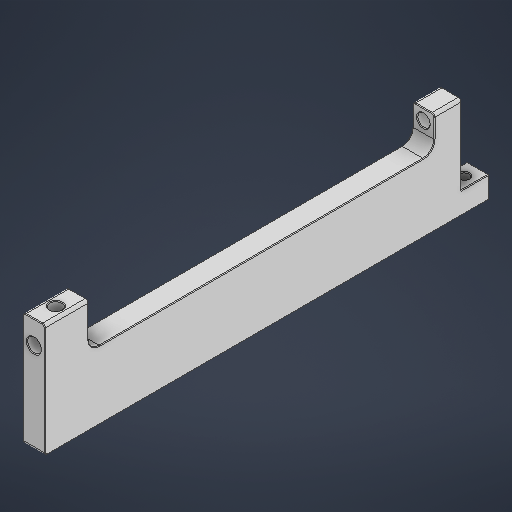
# Autodesk Inventor part: Half-Shaft-Motor
Saved by Autodesk Inventor 2025 (Build 290162010, 162A)
## iProperties
Created: 2025-12-05
Part Number: Half-Shaft-Motor
Material: Generic
Document SubType Name: Modeling
Designer: FizzyApple12
Density: 1 g/cm^3
Appearance: Default
Author: FizzyApple12
Autodesk Inventor part; units mm, degrees
ref_plane "YZ Plane" through (0, 0, 0) normal (1, 0, 0) x (0, 1, 0)
ref_plane "XZ Plane" through (0, 0, 0) normal (0, 1, 0) x (-1, 0, 0)
ref_plane "XY Plane" through (0, 0, 0) normal (0, 0, 1) x (1, 0, 0)
sketch "Sketch1" plane through (0, 0, 0) normal (0, 0, 1) x (1, 0, 0)
  circle A0 centre (0, 0) radius 2.5
  line L0 (-4, -8) -> (4, -8)
  line L1 (4, -8) -> (4, -33)
  line L2 (4, -33) -> (-4, -33)
  line L3 (-4, -33) -> (-4, -8)
  line L4 (0, 0) -> (0, -8) construction
  line L5 (-4, -8) -> (4, -8)
  line L6 (4, -8) -> (4, 4)
  line L7 (4, 4) -> (-4, 4)
  line L8 (-4, 4) -> (-4, -8)
  line L9 (0, 0) -> (0, 4) construction
  line L10 (-4, 4) -> (4, 4)
  line L11 (4, 4) -> (4, 8.5)
  line L12 (4, 8.5) -> (-4, 8.5)
  line L13 (-4, 8.5) -> (-4, 4)
  circle A1 centre (0, 0) radius 2.25
  line L14 (-4, -33) -> (4, -33)
  line L15 (4, -33) -> (4, -25)
  line L16 (4, -25) -> (-4, -25)
  line L17 (-4, -25) -> (-4, -33)
  point P0 (0, 2.5)
  dimension "d0" = 5
  dimension "d1" = 8
  dimension "d2" = 25
  dimension "d3" = 4
  dimension "d18" = 6
  dimension "d30" = 4.5
  dimension "d33" = 8
  dimension "d34" = 8
  constraints: 36 end point, 8 parallel, 4 horizontal, 4 perpendicular, 3 coincident, 2 midpoint, 2 point on line, 1 centre point, 1 vertical, 1 vertical alignment, 2 other
  measures "d1" distance of L1.end L2.end
  measures "d2" distance of L0.end L1.end
  measures "d3" distance of L4.start L9.end
  measures "d18" distance from line of L12 point (0, 2.5)
  measures "d30" diameter of A1
  measures "d33" distance from line of point (0, 0) L0
  measures "d34" distance of L15.end L14.end
extrude "Extrusion1" add sketch "Sketch1" against normal blind 16 contours L8 L7 L6 L0 | L0 L1 L16 L3 | L16 L1 L2 L3 | L13 L12 L11 L7
extrude "Extrusion2" add sketch "Sketch1" against normal blind 152.3335 contours L0 L1 L16 L3 | L16 L1 L2 L3
extrude "Extrusion3" add sketch "Sketch1" along normal blind 10 from surface at -152.3335 contours A0 | L8 L7 L6 L0 | L0 L1 L16 L3 | L16 L1 L2 L3 | A1
extrude "Extrusion5" add sketch "Sketch1" against normal blind 10 from surface at -152.3335 contours L16 L1 L2 L3
sketch "Sketch4" plane through (-4, -33, 0) normal (0, -1, 0) x (1, 0, 0)
  line L0 (0, -162.3335) -> (8, -162.3335) projected
  line L1 (0, -162.3335) -> (8, -162.3335)
  line L2 (8, -162.3335) -> (8, -152.3335)
  line L3 (8, -152.3335) -> (0, -152.3335)
  line L4 (0, -152.3335) -> (0, -162.3335)
  line L5 (0, -162.3335) -> (8, -152.3335) construction
  point P0 (4, 0)
  point P1 (4, -157.3335)
  dimension "d37" = 8
  dimension "d38" = 10
  constraints: 10 end point, 2 parallel, 1 horizontal, 1 midpoint, 1 perpendicular
  measures "d37" distance of L3.end L2.end
  measures "d38" distance of L2.end L1.end
hole "Hole3" at (0, -33, -157.3335) direction (0, 1, 0) diameter 3.4 end through all counterbore diameter 6.5 counterbore depth 3 clearance for "Socket Head Cap Screw" size "M3" standard "Ansi Metric M Profile"
sketch "Sketch2" plane through (0, 0, -152.3335) normal (0, 0, -1) x (-1, 0, 0)
  point P0 (0, 0)
  point P1 (0, 0)
hole "Hole1" at (0, 0, -152.3335) direction (0, 0, 1) diameter 4.5 depth 12 tip angle 118
sketch "Sketch3" plane through (-4, 8.5, 0) normal (0, 1, 0) x (1, 0, 0)
  line L0 (8, 0) -> (0, 0) construction
  line L1 (8, 0) -> (8, 16) construction
  line L2 (0, 16) -> (8, 16) construction
  line L3 (0, 0) -> (0, 16) construction
  line L4 (0, 0) -> (0, 16) construction
  line L5 (8, 16) -> (0, 0) construction
  point P0 (4, 0)
  point P1 (4, 8)
  constraints: 2 end point, 1 midpoint
hole "Hole2" at (0, 8.5, -8) direction (0, -1, 0) diameter 3.4 depth 9 tip angle 118 counterbore diameter 4.5 counterbore depth 5 clearance for "Socket Head Cap Screw" size "M3" standard "Ansi Metric M Profile"
extrude "Extrusion4" add sketch "Sketch1" against normal blind 0.5 from surface at -152.3335 contours A0
fillet "Fillet1" radius 4 2 edges at (0, -8, -16) (0, -8, -142.3335)
fillet "Fillet2" radius 1 5 edges at (4, 8.5, -8) (-4, 8.5, -8) (0, -33, 0) (4, 4, -147.3335) (-4, 4, -147.3335)
chamfer "Chamfer1" distance 0.25 angle 45 46 edges at (4, -11, -152.3335) (3.7071, 3.7071, -152.3335) (0, 4, -152.3335) (-3.7071, 3.7071, -152.3335) (-4, -11, -152.3335) (-4, -33, -81.6667) (-4, -32.7071, -0.2929) (-4, -12.25, 0) (-3.7071, 8.2071, 0) (0, 8.5, 0) (3.7071, 8.2071, 0) (4, -12.25, 0) (4, -32.7071, -0.2929) (4, -33, -81.6667) (0, -2.25, -142.3335) (4, -0.5, -142.3335) (3.7071, 3.7071, -142.3335) (0, 4, -142.3335) (-3.7071, 3.7071, -142.3335) (-4, -0.5, -142.3335) (-4, -6.8284, -141.1619) (-4, -8, -79.1667) (-4, -6.8284, -17.1716) (-4, 1.75, -16) (-3.7071, 8.2071, -16) (0, 8.5, -16) (3.7071, 8.2071, -16) (4, 1.75, -16) (4, -6.8284, -17.1716) (4, -8, -79.1667) (4, -6.8284, -141.1619) (-2.5, 0, -16) (-2.5, 0, 0) (0, 8.5, -10.25) (-0.0091, 2.5, -9.7) (0, 3.5, -9.7) (-2.5, 0, -152.3335) (4, -25, -157.3335) (-4, -25, -157.3335) (-4, -29, -162.3335) (0, -25, -162.3335) (4, -29, -162.3335) (0, -33, -162.3335) (0, -33, -154.0835) (0, -30, -155.6335) (0, -25, -155.6335)
body "Solid1"
